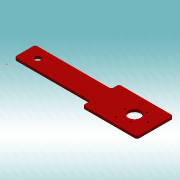
# Autodesk Inventor part: タイヤアーム
Saved by Autodesk Inventor 2015 (Build 190159000, 159)
## iProperties
Created: 2016-03-21
Part Number: タイヤアーム
Material: 一般
Document SubType Name: Modeling
Designer: buzztaka
Density: 1 g/cm^3
Appearance: 滑らか - 赤
Author: buzztaka
Autodesk Inventor part; units mm, degrees
ref_plane "YZ Plane" through (0, 0, 0) normal (1, 0, 0) x (0, 1, 0)
ref_plane "XZ Plane" through (0, 0, 0) normal (0, 1, 0) x (-1, 0, 0)
ref_plane "XY Plane" through (0, 0, 0) normal (0, 0, 1) x (1, 0, 0)
sketch "スケッチ1" plane through (0, 0, 0) normal (0, 0, 1) x (1, 0, 0)
  line L0 (0, 0) -> (252.35, 0)
  line L1 (252.35, 0) -> (252.35, 70)
  line L2 (252.35, 70) -> (0, 70)
  line L3 (0, 70) -> (0, 0)
  dimension "d0" = 70
  dimension "d1" = 252.35
  constraints: 8 end point, 2 parallel, 1 horizontal, 1 perpendicular
  measures "d0" distance of L2.end L0.start
  measures "d1" distance of L0.start L0.end
extrude "押し出し1" add sketch "スケッチ1" along normal blind 5
sketch "スケッチ2" plane through (0, 0, 5) normal (0, 0, 1) x (1, 0, 0)
  line L0 (0, 0) -> (252.35, 0) projected
  line L1 (0, 70) -> (0, 0) projected
  point P0 (25, 35)
  dimension "d4" = 35
  dimension "d5" = 25
  measures "d4" distance from line of L0 point (25, 35)
  measures "d5" distance from line of point (25, 35) L1
hole "穴1" at (25, 35, 5) direction (0, 0, -1) diameter 12 end through all
sketch "スケッチ3" plane through (0, 0, 5) normal (0, 0, 1) x (1, 0, 0)
  line L0 (252.35, 0) -> (252.35, 70) projected
  circle A0 centre (25, 35) radius 6 projected
  line L1 (0, 0) -> (252.35, 0) projected
  point P0 (212.35, 35)
  dimension "d14" = 187.35
  dimension "d15" = 35
  measures "d14" distance of A0.centre point (212.35, 35)
  measures "d15" distance from line of point (212.35, 35) L1
hole "穴2" at (212.35, 35, 5) direction (0, 0, -1) diameter 24 end through all
sketch "スケッチ4" plane through (0, 0, 5) normal (0, 0, 1) x (1, 0, 0)
  line L0 (252.35, 0) -> (252.35, 70) projected
  line L1 (0, 70) -> (0, 0) projected
  line L2 (252.35, 70) -> (0, 70) projected
  line L3 (0, 0) -> (252.35, 0) projected
  line L4 (0, 55) -> (147.35, 55)
  line L5 (0, 15) -> (147.35, 15)
  line L6 (147.35, 0) -> (147.35, 15)
  line L7 (147.35, 55) -> (147.35, 70)
  line L8 (147.35, 55) -> (0, 55)
  line L9 (0, 55) -> (0, 70)
  line L10 (0, 70) -> (147.35, 70)
  line L11 (147.35, 70) -> (147.35, 55)
  line L12 (147.35, 15) -> (0, 15)
  line L13 (0, 15) -> (0, 0)
  line L14 (0, 0) -> (147.35, 0)
  line L15 (147.35, 0) -> (147.35, 15)
  dimension "d24" = 15
  dimension "d25" = 15
  constraints: 24 end point, 5 parallel, 4 perpendicular, 2 horizontal, 2 point on line, 2 vertical
  measures "d24" distance from line of L2 L4.start
  measures "d25" distance from line of L3 L5.start
extrude "押し出し2" cut sketch "スケッチ4" against normal blind 10 contours L3 L1 L5 L6 | L7 L4 L1 L2
fillet "フィレット1" radius 4 2 edges at (147.35, 15, 2.5) (147.35, 55, 2.5)
sketch "スケッチ5" plane through (0, 0, 5) normal (0, 0, 1) x (1, 0, 0)
  line L0 (147.35, 0) -> (252.35, 0) projected
  circle A0 centre (212.35, 35) radius 12 projected
  point P0 (0, 0)
  point P1 (238.35, 35)
  point P2 (199.35, 57.5167)
  point P3 (199.35, 12.4833)
  dimension "d29" = 35
  dimension "d30" = 26
  dimension "d33" = 360
  constraints: 4 other
  measures "d29" distance from line of L0 point (238.35, 35)
  measures "d30" distance of A0.centre point (238.35, 35)
hole "穴3" at (238.35, 35, 5) at (199.35, 57.5167, 5) at (199.35, 12.4833, 5) direction (0, 0, -1) diameter 3.5 end through all
sketch "スケッチ6" plane through (0, 0, 5) normal (0, 0, 1) x (1, 0, 0)
  circle A0 centre (212.35, 35) radius 12 projected
  line L0 (147.35, 0) -> (252.35, 0) projected
  point P0 (0, 0)
  point P1 (194.35, 35)
  point P2 (221.35, 19.4115)
  point P3 (221.35, 50.5885)
  dimension "d42" = 18
  dimension "d43" = 35
  dimension "d46" = 360
  constraints: 4 other
  measures "d42" distance of A0.centre point (194.35, 35)
  measures "d43" distance from line of L0 point (194.35, 35)
hole "穴4" at (194.35, 35, 5) at (221.35, 19.4115, 5) at (221.35, 50.5885, 5) direction (0, 0, -1) diameter 3.5 end through all
fillet "フィレット2" radius 4 6 edges at (0, 55, 2.5) (0, 15, 2.5) (147.35, 0, 2.5) (147.35, 70, 2.5) (252.35, 70, 2.5) (252.35, 0, 2.5)
sketch "スケッチ7" plane through (0, 0, 0) normal (0, 0, -1) x (-1, 0, 0)
  point P0 (0, 0)
